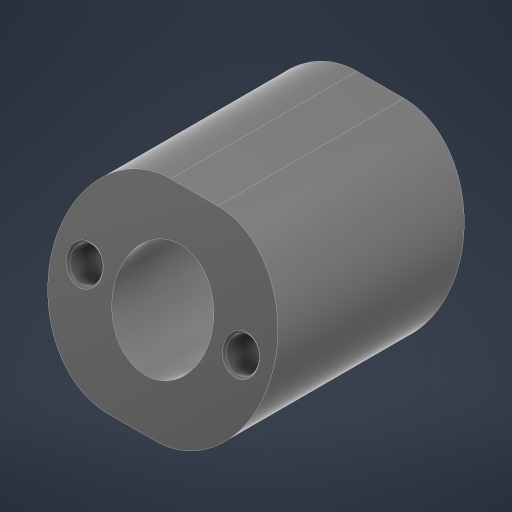
# Autodesk Inventor part: Leg_Loadpipe_Mount
Saved by Autodesk Inventor 2025 (Build 290162010, 162A)
## iProperties
Created: 2023-06-09
Part Number: Leg_Loadpipe_Mount
Material: Nylon 6/6
Document SubType Name: Modeling
Designer: dzw04
Density: 1.13 g/cm^3
Appearance: Smooth - Black
Author: dzw04
Autodesk Inventor part; units mm, degrees
ref_plane "YZ Plane" through (0, 0, 0) normal (1, 0, 0) x (0, 1, 0)
ref_plane "XZ Plane" through (0, 0, 0) normal (0, 1, 0) x (-1, 0, 0)
ref_plane "XY Plane" through (0, 0, 0) normal (0, 0, 1) x (1, 0, 0)
sketch "Sketch1" plane through (0, 0, 0) normal (1, 0, 0) x (0, 1, 0)
  line L0 (0, 0) -> (35.2385, -12.8258) construction
  line L1 (0, 0) -> (37.5, 0) construction
  line L2 (35.2385, -12.8258) -> (34.5544, -14.7051) construction
  line L3 (34.5544, -14.7051) -> (-0.684, -1.8794) construction
  line L4 (-0.684, -1.8794) -> (0, 0) construction
  line L5 (34.5544, -14.7051) -> (26.8932, -35.7543) construction
  line L6 (26.8932, -35.7543) -> (-8.3453, -22.9285) construction
  line L7 (-8.3453, -22.9285) -> (-9.0293, -24.8079) construction
  line L8 (-9.0293, -24.8079) -> (26.2091, -37.6336) construction
  line L9 (26.2091, -37.6336) -> (26.8932, -35.7543) construction
  line L10 (16.9352, -8.2923) -> (8.6633, -29.1191) construction
  line L11 (12.7992, 23.1416) -> (12.7992, -60.5529) construction
  line L12 (6.7992, 23.1416) -> (6.7992, -60.5529) construction
  line L13 (18.7992, 23.1416) -> (18.7992, -60.5529) construction
  line L14 (12.7992, -4.6585) -> (23.6057, -8.5918) construction
  line L15 (23.6057, -8.5918) -> (14.5764, -33.3997) construction
  line L16 (12.7992, -4.6585) -> (1.9928, -0.7253) construction
  line L17 (1.9928, -0.7253) -> (-7.0366, -25.5332) construction
  line L18 (1.7992, 23.1416) -> (1.7992, -60.5529)
  line L19 (23.7992, 23.1416) -> (23.7992, -60.5529)
  line L20 (18.9242, 23.1416) -> (18.9242, -60.5529)
  line L21 (6.6742, 23.1416) -> (6.6742, -60.5529)
  line L22 (1.7992, -2.7832) -> (6.6742, -4.5576)
  line L23 (1.7992, -26.6208) -> (6.6742, -28.3952)
  line L24 (23.7992, -34.6282) -> (18.9242, -32.8538)
  line L25 (23.7992, -10.7906) -> (18.9242, -9.0162)
  point P0 (12.7992, -18.7057)
  dimension "d1" = 37.5
  dimension "d2" = 20
  dimension "d3" = 2
  dimension "d4" = 22.4
  dimension "d5" = 37.5
  dimension "d6" = 2
  dimension "d7" = 6
  dimension "d8" = 6
  dimension "d9" = 11.5
  dimension "d10" = 11.5
  dimension "d13" = 11
  dimension "d14" = 11
  dimension "d15" = 4.875
  dimension "d16" = 4.875
  constraints: 52 end point, 24 point on line, 9 perpendicular, 6 parallel, 3 midpoint, 1 equal length, 1 horizontal, 1 vertical
  measures "d1" distance of L0.start L0.end
  measures "d2" angle of L0 L1
  measures "d3" distance of L0.end L2.end
  measures "d4" distance of L2.end L5.end
  measures "d5" distance of L5.end L6.end
  measures "d6" distance of L6.end L7.end
  measures "d7" distance between parallel lines of L11 L12
  measures "d8" distance between parallel lines of L13 L11
  measures "d9" distance of L14.start L14.end
  measures "d10" distance of L14.start L16.end
  measures "d13" distance between parallel lines of L11 L18
  measures "d14" distance between parallel lines of L11 L19
  measures "d15" distance between parallel lines of L19 L20
  measures "d16" distance between parallel lines of L18 L21
extrude "Extrusion1" add sketch "Sketch1" along normal blind 28
sketch "Sketch2" plane through (28, 0, 0) normal (1, 0, 0) x (0, 0, -1)
  line L0 (28.3952, 6.6742) -> (4.5576, 6.6742) projected
  line L1 (9.0162, 18.9242) -> (32.8538, 18.9242) projected
  line L2 (4.5576, 6.6742) -> (9.0162, 18.9242)
  line L3 (9.0162, 18.9242) -> (32.8538, 18.9242)
  line L4 (32.8538, 18.9242) -> (28.3952, 6.6742)
  line L5 (28.3952, 6.6742) -> (4.5576, 6.6742)
  point P0 (0, 0)
  point P1 (28.3952, 6.6742)
  constraints: 8 end point, 3 equal length
extrude "Extrusion2" add sketch "Sketch2" against normal blind 7.875
sketch "Sketch3" plane through (0, 0, 0) normal (-1, 0, 0) x (0, 0, 1)
  line L0 (-9.0162, 18.9242) -> (-32.8538, 18.9242) projected
  line L1 (-26.6208, 1.7992) -> (-28.3952, 6.6742) projected
  line L2 (-32.8538, 18.9242) -> (-28.3952, 6.6742)
  line L3 (-28.3952, 6.6742) -> (-4.5576, 6.6742)
  line L4 (-4.5576, 6.6742) -> (-9.0162, 18.9242)
  line L5 (-9.0162, 18.9242) -> (-32.8538, 18.9242)
  point P0 (0, 0)
  point P1 (-9.0162, 18.9242)
  constraints: 8 end point, 2 parallel, 1 collinear
extrude "Extrusion3" add sketch "Sketch3" against normal blind 7.875
fillet "Fillet1" radius 6.125 4 edges at (7.875, 6.6742, -16.4764) (20.125, 6.6742, -16.4764) (20.125, 18.9242, -20.935) (7.875, 18.9242, -20.935)
fillet "Fillet2" radius 11 4 edges at (0, 23.7992, -22.7094) (0, 1.7992, -14.702) (28, 1.7992, -14.702) (28, 23.7992, -22.7094)
sketch "Sketch4" plane through (11, 23.7992, -10.7906) normal (0, 0.3420201, 0.9396926) x (1, 0, 0)
  ellipse E0 centre (3, -11.706) end of major axis (3, -18.224) minor radius 6.125 construction
  circle A0 centre (3, -11.706) radius 10 construction
  circle A1 centre (-7, -11.706) radius 2
  circle A2 centre (13, -11.706) radius 2
  point P0 (-11, -26.0546)
  dimension "d25" = 20
  dimension "d26" = 4
  dimension "d27" = 4
  constraints: 3 centre point, 2 point on circle, 1 coincident, 1 other
  measures "d25" diameter of A0
  measures "d26" diameter of A1
  measures "d27" diameter of A2
extrude "Extrusion4" cut sketch "Sketch4" against normal blind 8
sketch "Sketch5" plane through (17, 1.7992, -26.6208) normal (0, -0.3420201, -0.9396926) x (-1, 0, 0)
  ellipse E0 centre (3, 11.706) end of major axis (3, 18.224) minor radius 6.125 projected
  circle A0 centre (3, 11.706) radius 10 construction
  circle A1 centre (-7, 11.706) radius 2
  circle A2 centre (13, 11.706) radius 2
  point P0 (17, -10.7956)
  dimension "d30" = 20
  dimension "d31" = 4
  dimension "d32" = 4
  constraints: 3 centre point, 2 point on circle, 1 coincident
  measures "d30" diameter of A0
  measures "d31" diameter of A1
  measures "d32" diameter of A2
extrude "Extrusion5" cut sketch "Sketch5" against normal blind 8 contours A1 | A2
sketch "Sketch6" plane through (11, 1.7992, -2.7832) normal (0, -1, 0) x (1, 0, 0)
  line L0 (0, -23.8376) -> (0, 0) projected
  line L1 (0, -11.9188) -> (6, -11.9188) construction
  line L2 (6, 0) -> (6, -23.8376) projected
  circle A0 centre (3, -11.9188) radius 2
  point P0 (-11, 2.7832)
  dimension "d35" = 4
  constraints: 3 midpoint, 2 end point, 1 centre point
  measures "d35" diameter of A0
extrude "Extrusion6" cut sketch "Sketch6" against normal blind 4.25
chamfer "Chamfer1" distance 0.25 angle 45 5 edges at (12, 1.7992, -14.702) (6, 12.7992, -30.6245) (26, 12.7992, -30.6245) (22, 12.7992, -6.7869) (2, 12.7992, -6.7869)
body "Solid1"
